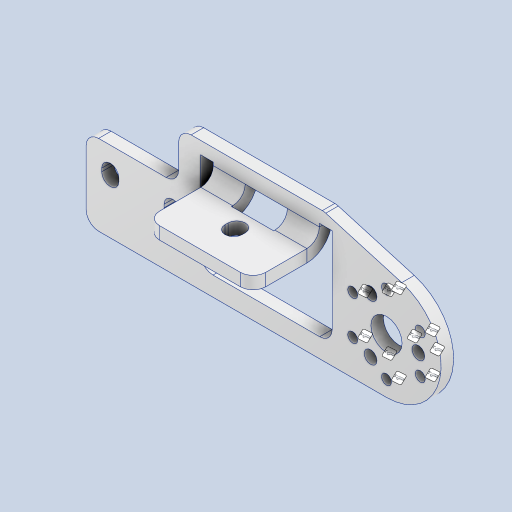
# Autodesk Inventor part: pitch_plate
Saved by Autodesk Inventor 2023 (Build 270158000, 158)
## iProperties
Created: 2024-12-05
Part Number: pitch_plate
Material: アルミニウム 5052
Document SubType Name: Sheet Metal
Designer: kiyo
Density: 2.68 g/cm^3
Sheet Metal Rule: Default_mm
Appearance: アルミニウム - フラット
Mass: 34.0559 g
Surface Area: 92.0836 cm^2
Volume: 12.7074 cm^3
Author: kiyo
Autodesk Inventor part; units mm, degrees
ref_plane "YZ Plane" through (0, 0, 0) normal (1, 0, 0) x (0, 1, 0)
ref_plane "XZ Plane" through (0, 0, 0) normal (0, 1, 0) x (-1, 0, 0)
ref_plane "XY Plane" through (0, 0, 0) normal (0, 0, 1) x (1, 0, 0)
sketch "スケッチ1" plane through (0, 0, 0) normal (1, 0, 0) x (0, 1, 0)
  arc A0 (0, -17.5) -> (4.891, 16.8026) centre (0, 0) ccw
  line L0 (-66.6, 24.048) -> (-20, 24.048)
  line L1 (0, -17.5) -> (-96.25, -17.5)
  line L2 (-96.25, -17.5) -> (-96.25, 8.25)
  line L3 (-20, 24.048) -> (4.891, 16.8026)
  line L4 (-17.4, 20.048) -> (-17.4, -11.35)
  line L5 (-17.4, -11.35) -> (-59.6, -11.35)
  line L6 (-59.6, -11.35) -> (-59.6, 20.048)
  line L7 (-88.5, 0.5) -> (-88.5, -0.5) construction
  line L8 (-85.75, 0.5) -> (-85.75, -0.5)
  line L9 (-91.25, -0.5) -> (-91.25, 0.5)
  arc A1 (-85.75, 0.5) -> (-91.25, 0.5) centre (-88.5, 0.5) ccw
  arc A2 (-91.25, -0.5) -> (-85.75, -0.5) centre (-88.5, -0.5) ccw
  line L10 (-68.5, 0.5) -> (-68.5, -0.5) construction
  line L11 (-65.75, 0.5) -> (-65.75, -0.5)
  line L12 (-71.25, -0.5) -> (-71.25, 0.5)
  arc A3 (-65.75, 0.5) -> (-71.25, 0.5) centre (-68.5, 0.5) ccw
  arc A4 (-71.25, -0.5) -> (-65.75, -0.5) centre (-68.5, -0.5) ccw
  circle A5 centre (0, 0) radius 5
  circle A6 centre (10.2, 0) radius 2.05
  circle A7 centre (-5.1, 8.8335) radius 2.05
  circle A8 centre (-5.1, -8.8335) radius 2.05
  line L13 (-21.5, 20.048) -> (-21.5, -7.25)
  line L14 (-21.5, -7.25) -> (-55.5, -7.25)
  line L15 (-55.5, -7.25) -> (-55.5, 20.048)
  line L16 (-59.6, 20.048) -> (-55.5, 20.048)
  line L17 (-21.5, 20.048) -> (-17.4, 20.048)
  line L18 (-66.6, 24.048) -> (-66.6, 8.25)
  line L19 (-66.6, 8.25) -> (-96.25, 8.25)
  line L20 (-38.5, 3.5) -> (-38.5, 4.5) construction
  line L21 (-35.75, 3.5) -> (-35.75, 4.5)
  line L22 (-41.25, 4.5) -> (-41.25, 3.5)
  arc A9 (-41.25, 3.5) -> (-35.75, 3.5) centre (-38.5, 3.5) ccw
  arc A10 (-35.75, 4.5) -> (-41.25, 4.5) centre (-38.5, 4.5) ccw
  line L23 (-45.25, 19.048) -> (-31.75, 19.048)
  line L24 (-31.75, 9.598) -> (-45.25, 9.598)
  line L25 (-45.25, 9.598) -> (-45.25, 19.048)
  line L26 (-31.75, 19.048) -> (-31.75, 9.598)
  point P0 (-88.5, 0)
  point P1 (-68.5, 0)
  point P2 (-65.75, 0)
  point P3 (-71.25, 0)
  point P4 (-38.5, 4)
  point P5 (-41.25, 4)
  point P6 (-35.75, 4)
  point P7 (-38.5, -7.25)
  point P8 (-38.5, 0.75)
  point P9 (-45.25, 14.323)
  point P10 (-88.5, 3.25)
  point P11 (-91.25, 0)
  dimension "d0" = 35
  dimension "d2" = 20
  dimension "d6" = 5.5
  dimension "d7" = 1
  dimension "d8" = 1
  dimension "d9" = 5.5
  dimension "d10" = 0
  dimension "d12" = 20
  dimension "d14" = 10.2
  dimension "d15" = 4.1
  dimension "d16" = 0
  dimension "d20" = 10
  dimension "d27" = 360
  dimension "d30" = 4.1
  dimension "d55" = 4.1
  dimension "d72" = 5.5
  dimension "d73" = 1
  dimension "d74" = 0
  dimension "d79" = 30
  dimension "d97" = 4
  dimension "d98" = 16.048
  dimension "d99" = 4
  dimension "d100" = 0
  dimension "d102" = 17.4
  dimension "d103" = 8
  dimension "d105" = 9.45
  dimension "d107" = 13.5
  dimension "d108" = 5
  dimension "d109" = 6.75
  dimension "d122" = 17
  dimension "d124" = 7
  dimension "d125" = 5
  dimension "d126" = 5
  measures "d0" diameter of A0
  measures "d2" horizontal distance of L0.end point (0, 0)
  measures "d6" distance between parallel lines of L9 L8
  measures "d7" distance of L8.start L8.end
  measures "d8" distance of L12.start L12.end
  measures "d9" distance of point (-65.75, 0) point (-71.25, 0)
  measures "d10" vertical distance of point (-88.5, 0) point (-68.5, 0)
  measures "d12" distance of point (-88.5, 0) point (-68.5, 0)
  measures "d14" distance of point (0, 0) A6.centre
  measures "d15" diameter of A6
  measures "d16" vertical distance of point (0, 0) A6.centre
  measures "d20" diameter of A5
  measures "d30" distance of L13.start L4.start
  measures "d55" distance between parallel lines of L5 L14
  measures "d72" distance of point (-41.25, 4) point (-35.75, 4)
  measures "d73" distance of L21.start L21.end
  measures "d74" horizontal distance of point (-38.5, -7.25) point (-38.5, 4)
  measures "d79" horizontal distance of point (-68.5, 0) point (-38.5, 4)
  measures "d97" vertical distance of point (-68.5, 0) point (-38.5, 4)
  measures "d98" distance from line of L17 point (-38.5, 4)
  measures "d99" distance between parallel lines of L16 L0
  measures "d100" vertical distance of point (0, 0) point (-68.5, 0)
  measures "d102" distance from line of A5.centre L4
  measures "d103" distance from line of point (-38.5, 0.75) L14
  measures "d105" distance of L24.end L23.start
  measures "d107" distance of L23.start L23.end
  measures "d108" distance between parallel lines of L23 L0
  measures "d109" distance from line of point (-38.5, 4) L25
  measures "d122" horizontal distance of L15.end point (-38.5, 4)
  measures "d124" distance between parallel lines of L18 L6
  measures "d125" distance from line of point (-88.5, 3.25) L19
  measures "d126" distance from line of point (-91.25, 0) L2
extrude "プレート1" add sketch "スケッチ1" along normal blind 4
sketch "スケッチ5" plane through (4, 0, 0) normal (1, 0, 0) x (0, 0, -1)
  line L0 (-20.048, -55.5) -> (7.25, -55.5) projected
  line L1 (-19.048, -55.5) -> (-19.048, -21.5)
  line L2 (7.25, -21.5) -> (-20.048, -21.5) projected
  line L3 (-20.048, -59.6) -> (-20.048, -55.5) projected
  point P0 (0, 0)
  dimension "d64" = 1
  constraints: 2 end point, 2 point on line, 1 vertical
  measures "d64" distance between parallel lines of L1 L3
fold "折り曲げ4" angle 90 bend radius 4 thickness 4 k factor 0.44 line from (4, -55.5, 19.048) to (4, -21.5, 19.048) line at bend start moving side (0, 0, -1) folds toward (1, 0, 0)
fillet "フィレット1" radius 4 9 edges at (2, -66.6, 24.048) (2, -20, 24.048) (2, -66.6, 8.25) (2, -96.25, 8.25) (2, -96.25, -17.5) (25.2502, -55.5, 13.048) (25.2502, -21.5, 13.048) (2, -59.6, -11.35) (2, -17.4, -11.35)
sketch "スケッチ6" plane through (4, 0, 0) normal (1, 0, 0) x (0, 0, -1)
  circle A0 centre (0, 0) radius 5 projected
  point P0 (-12.5, 0)
  point P1 (-6.25, -10.8253)
  point P2 (6.25, -10.8253)
  point P3 (12.5, 0)
  point P4 (6.25, 10.8253)
  point P5 (-6.25, 10.8253)
  dimension "d83" = 12.5
  dimension "d84" = 0
  dimension "d87" = 360
  constraints: 7 other
  measures "d83" distance of point (0, 0) point (-12.5, 0)
  measures "d84" vertical distance of point (0, 0) point (-12.5, 0)
hole "穴1" at (4, 0, 12.5) at (4, -10.8253, 6.25) at (4, -10.8253, -6.25) at (4, 0, -12.5) at (4, 10.8253, -6.25) at (4, 10.8253, 6.25) direction (-1, 0, 0) diameter 3.2 depth 4
equation "\"BendRadius\" = Thickness"
equation "\"BendReliefWidth\" = Thickness"
equation "\"BendReliefDepth\" = 0.5 * Thickness"
equation "\"CornerReliefSize\" = 4 * Thickness"
equation "\"MinimumRemnant\" = 2 * Thickness"
equation "\"TransitionRadius\" = BendRadius"
equation "\"JacobiRadiusSize\" = BendRadius"
equation "\"GapSize\" = Thickness"
